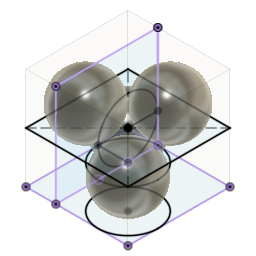
n=4_ryoji.jp (Autodesk Fusion 360 design; units mm, degrees)
Autodesk Fusion 360 part; units mm, degrees
sketch "スケッチ1" plane through (0, 0, 0) normal (0, 0, 1) x (1, 0, 0) in component "Component"
  line L0 (50, -50) -> (-50, -50)
  line L1 (-50, -50) -> (-50, 50)
  line L2 (-50, 50) -> (50, 50)
  line L3 (50, 50) -> (50, -50)
  line L4 (50, -50) -> (-50, 50) construction
  line L5 (-50, -50) -> (50, 50) construction
  dimension "d14" = 100
  dimension "d15" = 100
  constraint perpendicular L0 L1
  constraint parallel L0 L2
  constraint parallel L1 L3
  constraint horizontal L0
  constraint coincident L4 origin
  constraint coincident L5 origin
  measures "d14" distance of L1.end L2.end
  measures "d15" distance of L0.end L1.end
extrude "押し出し1" add sketch "スケッチ1" along normal mid plane 100 makes body 1 in component "Component"
offset_surface "サーフェス オフセット1" offset 0 6 faces at (-50, -16.6667, -16.6667) (-16.6667, -16.6667, -50) (-16.6667, 50, -16.6667) (-16.6667, -16.6667, 50) (-16.6667, -50, 16.6667) (50, -16.6667, 16.6667) on bodies 1 makes body 2 in component "Component"
delete_body "RemoveBody1" bodies 1 in component "Component"
sketch "スケッチ2" plane through (0, 0, -50) normal (0, 0, -1) x (1, 0, 0) in component "Component"
  circle A0 centre (-20.7107, -20.7107) radius 29.2893
  circle A1 centre (20.7107, 20.7107) radius 29.2893
  line L0 (50, -50) -> (-50, -50)
  line L1 (-50, -50) -> (-50, 50)
  line L2 (50, 50) -> (50, -50)
  line L3 (-50, 50) -> (50, 50)
  line L4 (-20.7107, -20.7107) -> (-50, -20.7107)
  constraint tangent A0 L0
  constraint tangent A0 L1
  constraint tangent A1 L2
  constraint tangent A1 L3
  constraint equal A0 A1
  constraint coincident A0.centre L4.start
  constraint coincident L1 L4.end
  constraint coincident A0 L4.end
  constraint perpendicular L1 L4
  constraint tangent A0 A1
ref_plane "作業平面3" through (-20.7107, 0, 0) normal (-1, 0, 0) x (0, -1, 0) in component "Component"
sketch "スケッチ4" plane through (-20.7107, 0, 0) normal (-1, 0, 0) x (0, 1, 0) in component "Component"
  line L0 (50, 50) -> (50, -50)
  line L1 (50, -50) -> (50, 50)
  line L2 (50, 50) -> (50, -50)
  line L3 (50, -50) -> (-50, -50)
  line L4 (-50, -50) -> (-50, 50)
  line L5 (-50, 50) -> (50, 50)
  circle A0 centre (20.7107, 20.7107) radius 29.2893
  line L6 (50, 50) -> (-8.5786, 50)
  line L7 (-8.5786, 20.7107) -> (50, 20.7107)
  point P0 (20.7107, 50)
  constraint tangent L2 A0
  constraint tangent A0 L6
  constraint vertical P0 A0.centre
  constraint coincident L1 L7.end
  constraint coincident A0 L7.end
  constraint perpendicular L1 L7
  constraint coincident A0 L7.start
revolve "回転2" add sketch "スケッチ4" angle 360 about axis through (-20.7107, -8.5786, -20.7107) along (0, 1, 0) separate body contours A0 L7 picked at (16.5556, 30.9809) makes body 3 in component "Component"
ref_plane "作業平面4" through (-50, -50, -50) normal (0.707107, -0.707107, 0) x (0.707107, 0.707107, 0) in component "Component"
mirror "ミラー3" about plane through (-50, -50, -50) normal (0.707107, -0.707107, 0) of bodies 3 makes body 4 in component "Component"
mirror "ミラー4" about plane through (0, 0, 0) normal (0, 0, 1) of bodies 3 4 makes body 5 at (4.4376, 16.8877, 35.2301) makes body 6 at (16.8877, 4.4376, 6.1913) in component "Component"
move_body "移動2" bodies 5 6 to x (0, 1, 0) y (-1, 0, 0) z (0, 0, 1) at (0, 0, 0) in component "Component"
component "Component" placed x (1, 0, 0) y (0, 1, 0) z (0, 0, 1) at (0, 0, 0)
equation "rr = 30 mm"
